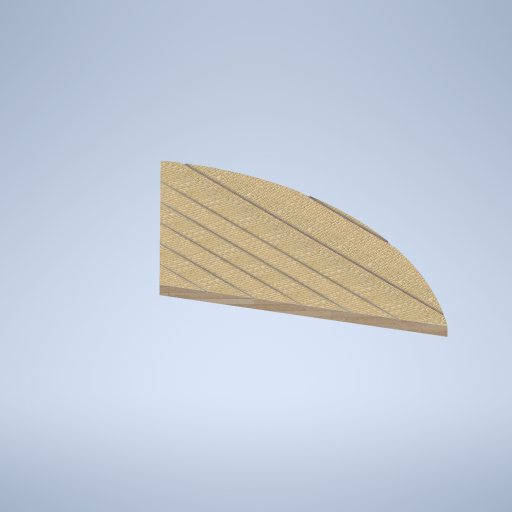
# Autodesk Inventor part: eave_panel_corner
Saved by Autodesk Inventor 2024.2 (Build 282272000, 272)
## iProperties
Created: 2024-05-24
Part Number: eave_panel_corner
Material: Wood (Maple)
Document SubType Name: Modeling
Designer: LOSTER_1
Density: 0.67 g/cm^3
Appearance: Natural Maple - Glossy Dark Tint
Author: LOSTER_1
Autodesk Inventor part; units mm, degrees
ref_plane "YZ Plane" through (0, 0, 0) normal (1, 0, 0) x (0, 1, 0)
ref_plane "XY Plane" through (0, 0, 0) normal (0, 0, 1) x (1, 0, 0)
sketch "Sketch1" plane through (0, 0, 0) normal (0, 1, 0) x (-1, 0, 0)
  arc A0 (-1548.1484, -783.8336) -> (1537.1126, -783.8336) centre (-5.5179, 1309.0809) ccw
  line L0 (6.8713, 758.7471) -> (-1548.1484, -783.8336)
  line L1 (1537.1126, -783.8336) -> (6.8713, 758.7471)
  line L2 (-1548.1484, -783.8336) -> (1537.1126, -783.8336)
  point P0 (0, 0)
  point P1 (-841.7636, 217.1232)
  constraints: 6 end point, 2 point on circle, 1 centre point, 1 horizontal
ref_plane "Work Plane1" through (-6.8713, 0, 758.7471) normal (0.7042616, 0, 0.7099406) x (0.7099406, 0, -0.7042616)
ref_plane "Work Plane2" through (-1537.1126, 0, -783.8336) normal (-0.7099406, 0, 0.7042616) x (0.7042616, 0, 0.7099406)
ref_plane "Work Plane3" through (-6.8713, 0, 758.7471) normal (0, -1, 0) x (0.7099406, 0, -0.7042616)
extrude "Extrusion1" add sketch "Sketch1" along normal blind 100 contours L2 A0
sketch "Sketch2" plane through (-1537.1126, 0, -783.8336) normal (-0.7099406, 0, 0.7042616) x (0.7042616, 0, 0.7099406)
  line L0 (0, 0) -> (0, 100) projected
  line L1 (0, 100) -> (0, 0)
  line L2 (0, 0) -> (2172.8308, 383.1287)
  line L3 (0, 0) -> (2206.3502, 0) construction
  line L4 (0, 100) -> (2172.8308, 483.1287)
  line L5 (0, 100) -> (2206.3502, 100) construction
  line L6 (2172.8308, 483.1287) -> (2172.8308, 383.1287)
  point P0 (1639.0046, 0)
  dimension "d4" = 10
  dimension "d5" = 10
  constraints: 12 end point, 2 equal length, 2 horizontal
  measures "d4" angle of L3 L2
  measures "d5" angle of L5 L4
sketch "Sketch4" plane through (-6.8713, 0, 758.7471) normal (0.7042616, 0, 0.7099406) x (0.7099406, 0, -0.7042616)
  line L0 (0, 483.1287) -> (0, 383.1287) projected
  line L1 (0, 483.1287) -> (0, 383.1287)
  line L2 (2190.3519, 0) -> (0, 0) projected
  line L3 (2190.3519, 0) -> (0, 383.1287)
  line L4 (2190.3519, 0) -> (2190.3519, 100) projected
  line L5 (2190.3519, 0) -> (2190.3519, 100)
  line L6 (2190.3519, 100) -> (0, 483.1287)
  point P0 (539.2347, 0)
  constraints: 8 end point, 2 collinear
loft "Loft1" add profiles "Sketch4", "Sketch2"
sketch "Sketch5" plane through (-6.8713, 0, 758.7471) normal (0.7042616, 0, 0.7099406) x (0.7099406, 0, -0.7042616)
  line L0 (344.7656, 422.8235) -> (344.7656, 412.8601)
  line L1 (344.7656, 422.8235) -> (364.2941, 419.4076)
  line L2 (364.2941, 419.4076) -> (364.2941, 409.4443)
  line L3 (364.2941, 409.4443) -> (344.7656, 412.8601)
  point P0 (539.2347, 0)
  constraints: 8 end point, 2 vertical, 1 parallel
sketch "Sketch6" plane through (-1537.1126, 0, -783.8336) normal (-0.7099406, 0, 0.7042616) x (0.7042616, 0, 0.7099406)
  line L0 (1828.1481, 422.3518) -> (1828.1481, 412.4389)
  line L1 (1828.1481, 412.4389) -> (1808.7176, 409.0128)
  line L2 (1808.7176, 409.0128) -> (1808.7176, 418.9257)
  line L3 (1808.7176, 418.9257) -> (1828.1481, 422.3518)
  point P0 (1639.0046, 0)
  constraints: 8 end point, 2 parallel, 1 vertical
loft "Loft2" cut profiles "Sketch6", "Sketch5"
sketch "Sketch8" plane through (-1537.1126, 0, -783.8336) normal (-0.7099406, 0, 0.7042616) x (0.7042616, 0, 0.7099406)
  line L0 (1464.0348, 358.1488) -> (1464.0348, 347.7426)
  line L1 (1464.0348, 347.7426) -> (1444.0611, 344.2207)
  line L2 (1444.0611, 344.2207) -> (1444.0611, 354.6269)
  line L3 (1444.0611, 354.6269) -> (1464.0348, 358.1488)
  point P0 (1639.0046, 0)
  constraints: 8 end point, 1 parallel, 1 vertical
sketch "Sketch10" plane through (-6.8713, 383.1287, 758.7471) normal (0.7042616, 0, 0.7099406) x (0.7099406, 0, -0.7042616)
  line L0 (709.0597, -24.0262) -> (709.0597, -34.0321)
  line L1 (709.0597, -34.0321) -> (728.8357, -37.4913)
  line L2 (728.8357, -37.4913) -> (728.8357, -27.4854)
  line L3 (709.0597, -24.0262) -> (728.8357, -27.4854)
  point P0 (539.2347, -383.1287)
  constraints: 8 end point, 2 parallel, 1 vertical
loft "Loft3" cut profiles "Sketch10", "Sketch8"
sketch "Sketch11" plane through (-1537.1126, 0, -783.8336) normal (-0.7099406, 0, 0.7042616) x (0.7042616, 0, 0.7099406)
  line L0 (1099.3784, 293.8501) -> (1099.3784, 283.8797)
  line L1 (1099.3784, 283.8797) -> (1079.8614, 280.4384)
  line L2 (1079.8614, 280.4384) -> (1079.8614, 290.4087)
  line L3 (1079.8614, 290.4087) -> (1099.3784, 293.8501)
  point P0 (1639.0046, 0)
  point P1 (1444.0611, 354.6269)
  constraints: 8 end point, 2 parallel, 1 vertical
sketch "Sketch12" plane through (-6.8713, 383.1287, 758.7471) normal (0.7042616, 0, 0.7099406) x (0.7099406, 0, -0.7042616)
  line L0 (1073.6012, -87.7906) -> (1073.6012, -97.6756)
  line L1 (1073.6012, -97.6756) -> (1092.8187, -101.037)
  line L2 (1092.8187, -101.037) -> (1092.8187, -91.152)
  line L3 (1073.6012, -87.7906) -> (1092.8187, -91.152)
  point P0 (539.2347, -383.1287)
  constraints: 8 end point, 1 parallel, 1 vertical
loft "Loft4" cut profiles "Sketch12", "Sketch11"
sketch "Sketch13" plane through (-1537.1126, 0, -783.8336) normal (-0.7099406, 0, 0.7042616) x (0.7042616, 0, 0.7099406)
  line L0 (1079.8614, 280.4384) -> (1079.8614, 290.4087) projected
  line L1 (735.1787, 229.6318) -> (735.1787, 219.9385)
  line L2 (735.1787, 219.9385) -> (715.8629, 216.5326)
  line L3 (715.8629, 216.5326) -> (715.8629, 226.2259)
  line L4 (735.1787, 229.6318) -> (715.8629, 226.2259)
  point P0 (1639.0046, 0)
  constraints: 8 end point, 2 parallel, 1 vertical
sketch "Sketch14" plane through (-6.8713, 383.1287, 758.7471) normal (0.7042616, 0, 0.7099406) x (0.7099406, 0, -0.7042616)
  line L0 (1437.5842, -151.4572) -> (1437.5842, -161.5841)
  line L1 (1437.5842, -161.5841) -> (1457.5803, -165.0817)
  line L2 (1457.5803, -165.0817) -> (1457.5803, -154.9548)
  line L3 (1437.5842, -151.4572) -> (1457.5803, -154.9548)
  point P0 (539.2347, -383.1287)
  constraints: 8 end point, 1 parallel, 1 vertical
loft "Loft5" cut profiles "Sketch13", "Sketch14"
sketch "Sketch15" plane through (-6.8713, 383.1287, 758.7471) normal (0.7042616, 0, 0.7099406) x (0.7099406, 0, -0.7042616)
  line L0 (1802.3459, -215.26) -> (1802.3459, -225.0779)
  line L1 (1802.3459, -225.0779) -> (1822.2998, -228.5682)
  line L2 (1822.2998, -228.5682) -> (1822.2998, -218.7503)
  line L3 (1822.2998, -218.7503) -> (1802.3459, -215.26)
  point P0 (539.2347, -383.1287)
  constraints: 8 end point, 1 parallel, 1 vertical
sketch "Sketch16" plane through (-1537.1126, 0, -783.8336) normal (-0.7099406, 0, 0.7042616) x (0.7042616, 0, 0.7099406)
  line L0 (371.1802, 165.4491) -> (371.1802, 155.7332)
  line L1 (371.1802, 155.7332) -> (351.2645, 152.2215)
  line L2 (351.2645, 152.2215) -> (351.2645, 161.9374)
  line L3 (371.1802, 165.4491) -> (351.2645, 161.9374)
  point P0 (1639.0046, 0)
  constraints: 8 end point, 1 parallel, 1 vertical
loft "Loft6" cut profiles "Sketch16", "Sketch15"
ref_plane "Work Plane4" through (-1537.1126, 0, -783.8336) normal (0.9999919, 0, 0.0040156) x (0, 1, 0)
sketch "Sketch17" plane through (-1537.1126, 0, -783.8336) normal (0.9999919, 0, 0.0040156) x (0, 1, 0)
  line L0 (100, -513.297) -> (100, 0) projected
  line L1 (0, -513.297) -> (100, -513.297) projected
  line L2 (0, -513.297) -> (0, 0) projected
  line L3 (0, 0) -> (100, 0) projected
  line L4 (100, -478.6501) -> (90.1043, -478.6501)
  line L5 (90.1043, -478.6501) -> (90.1043, -458.6515)
  line L6 (90.1043, -458.6515) -> (100, -458.6515)
  line L7 (100, -478.6501) -> (100, -458.6515)
  line L8 (100, -458.6515) -> (100, -108.4646)
  line L9 (100, -108.4646) -> (90.1043, -108.4646)
  line L10 (90.1043, -108.4646) -> (90.1043, -88.0516)
  line L11 (90.1043, -88.0516) -> (100, -88.0516)
  line L12 (100, -108.4646) -> (100, -88.0516)
  point P0 (0, 777.6548)
  point P1 (100, -12.3893)
  point P2 (0, -12.3893)
  constraints: 18 end point, 6 perpendicular, 6 point on line, 1 collinear
extrude "Extrusion2" cut sketch "Sketch17" along normal through all contours L4 L5 L6 L0 | L9 L10 L11 L0
body "Solid1"
